Autodesk Fusion 360 part; units mm, degrees
(part 9 of 18)
  line L6113 (198.6347, -76.3898) -> (199.6463, -76.3898)
  line L6114 (199.6463, -76.3898) -> (199.6463, -77.3314)
  line L6115 (198.6347, -77.3314) -> (198.6347, -76.3898)
  line L6116 (199.6463, -77.3314) -> (198.6347, -77.3314)
  line L6117 (195.3245, -57.327) -> (196.3361, -57.327)
  line L6118 (196.3361, -58.2686) -> (195.3245, -58.2686)
  line L6119 (195.3245, -58.2686) -> (195.3245, -57.327)
  line L6120 (196.3361, -57.327) -> (196.3361, -58.2686)
  line L6121 (198.6347, -57.327) -> (199.6463, -57.327)
  line L6122 (199.6463, -58.2686) -> (198.6347, -58.2686)
  line L6123 (198.6347, -58.2686) -> (198.6347, -57.327)
  line L6124 (199.6463, -57.327) -> (199.6463, -58.2686)
  line L6125 (196.3361, -19.2142) -> (196.3361, -20.1558)
  line L6126 (195.3245, -20.1558) -> (195.3245, -19.2142)
  line L6127 (196.3361, -20.1558) -> (195.3245, -20.1558)
  line L6128 (195.3245, -19.2142) -> (196.3361, -19.2142)
  line L6129 (198.6347, -20.1558) -> (198.6347, -19.2142)
  line L6130 (199.6463, -19.2142) -> (199.6463, -20.1558)
  line L6131 (199.6463, -20.1558) -> (198.6347, -20.1558)
  line L6132 (198.6347, -19.2142) -> (199.6463, -19.2142)
  line L6133 (202.1892, -3.3092) -> (202.1892, -4.3108)
  line L6134 (201.2876, -4.3108) -> (201.2876, -3.3092)
  line L6135 (201.2876, -3.3092) -> (202.1892, -3.3092)
  line L6136 (202.1892, -4.3108) -> (201.2876, -4.3108)
  line L6137 (203.5892, -4.3108) -> (202.6876, -4.3108)
  line L6138 (202.6876, -4.3108) -> (202.6876, -3.3092)
  line L6139 (202.6876, -3.3092) -> (203.5892, -3.3092)
  line L6140 (203.5892, -3.3092) -> (203.5892, -4.3108)
  line L6141 (199.3826, -7.2318) -> (199.3826, -6.2302)
  line L6142 (200.2842, -7.2318) -> (199.3826, -7.2318)
  line L6143 (200.2842, -6.2302) -> (200.2842, -7.2318)
  line L6144 (199.3826, -6.2302) -> (200.2842, -6.2302)
  line L6145 (201.6842, -6.2302) -> (201.6842, -7.2318)
  line L6146 (201.6842, -7.2318) -> (200.7826, -7.2318)
  line L6147 (200.7826, -6.2302) -> (201.6842, -6.2302)
  line L6148 (200.7826, -7.2318) -> (200.7826, -6.2302)
  line L6149 (205.9896, -5.3268) -> (205.9896, -4.3252)
  line L6150 (206.8912, -4.3252) -> (206.8912, -5.3268)
  line L6151 (205.9896, -4.3252) -> (206.8912, -4.3252)
  line L6152 (206.8912, -5.3268) -> (205.9896, -5.3268)
  line L6153 (205.4912, -4.3252) -> (205.4912, -5.3268)
  line L6154 (204.5896, -4.3252) -> (205.4912, -4.3252)
  line L6155 (204.5896, -5.3268) -> (204.5896, -4.3252)
  line L6156 (205.4912, -5.3268) -> (204.5896, -5.3268)
  arc A664 (8.7123, -8.0011) -> (10.6139, -8.0011) centre (9.6631, -8.0011) ccw
  line L6157 (10.6139, -8.0011) -> (10.6139, -8.0011)
  arc A665 (10.6139, -8.0011) -> (8.7123, -8.0011) centre (9.6631, -8.0011) ccw
  arc A666 (8.7123, -5.4611) -> (10.6139, -5.4611) centre (9.6631, -5.4611) ccw
  arc A667 (10.6139, -5.4611) -> (8.7123, -5.4611) centre (9.6631, -5.4611) ccw
  line L6158 (10.6139, -5.4611) -> (10.6139, -5.4611)
  arc A668 (8.7123, -2.9211) -> (10.6139, -2.9211) centre (9.6631, -2.9211) ccw
  line L6159 (10.6139, -2.9211) -> (10.6139, -2.9211)
  arc A669 (10.6139, -2.9211) -> (8.7123, -2.9211) centre (9.6631, -2.9211) ccw
  arc A670 (-5.7879, -8.0011) -> (-3.8863, -8.0011) centre (-4.8371, -8.0011) ccw
  arc A671 (-3.8863, -8.0011) -> (-5.7879, -8.0011) centre (-4.8371, -8.0011) ccw
  arc A672 (-3.8863, -2.9211) -> (-5.7879, -2.9211) centre (-4.8371, -2.9211) ccw
  arc A673 (-5.7879, -2.9211) -> (-3.8863, -2.9211) centre (-4.8371, -2.9211) ccw
  line L6160 (1.3129, 1.2398) -> (3.0129, 1.2398)
  line L6161 (4.1223, -0.4205) -> (3.862, -0.8101)
  line L6162 (3.4725, 1.1484) -> (3.862, 0.8881)
  line L6163 (4.2137, 0.039) -> (4.1223, -0.4205)
  line L6164 (3.4725, -1.0704) -> (3.0129, -1.1618)
  line L6165 (0.1121, 0.039) -> (0.2035, 0.4985)
  line L6166 (0.8534, 1.1484) -> (1.3129, 1.2398)
  line L6167 (3.862, -0.8101) -> (3.4725, -1.0704)
  line L6168 (0.4638, -0.8101) -> (0.2035, -0.4205)
  line L6169 (0.4638, 0.8881) -> (0.8534, 1.1484)
  line L6170 (1.3129, -1.1618) -> (0.8534, -1.0704)
  line L6171 (0.2035, 0.4985) -> (0.4638, 0.8881)
  line L6172 (3.0129, -1.1618) -> (1.3129, -1.1618)
  line L6173 (3.0129, 1.2398) -> (3.4725, 1.1484)
  line L6174 (0.2035, -0.4205) -> (0.1121, 0.039)
  line L6175 (4.1223, 0.4985) -> (4.2137, 0.039)
  line L6176 (0.8534, -1.0704) -> (0.4638, -0.8101)
  line L6177 (3.862, 0.8881) -> (4.1223, 0.4985)
  line L6178 (3.4725, -9.8516) -> (3.862, -10.1119)
  line L6179 (1.3129, -9.7602) -> (3.0129, -9.7602)
  line L6180 (0.4638, -10.1119) -> (0.8534, -9.8516)
  line L6181 (3.0129, -12.1618) -> (1.3129, -12.1618)
  line L6182 (0.1121, -10.961) -> (0.2035, -10.5015)
  line L6183 (3.862, -10.1119) -> (4.1223, -10.5015)
  line L6184 (4.2137, -10.961) -> (4.1223, -11.4205)
  line L6185 (0.4638, -11.8101) -> (0.2035, -11.4205)
  line L6186 (4.1223, -10.5015) -> (4.2137, -10.961)
  line L6187 (3.4725, -12.0704) -> (3.0129, -12.1618)
  line L6188 (3.0129, -9.7602) -> (3.4725, -9.8516)
  line L6189 (1.3129, -12.1618) -> (0.8534, -12.0704)
  line L6190 (4.1223, -11.4205) -> (3.862, -11.8101)
  line L6191 (3.862, -11.8101) -> (3.4725, -12.0704)
  line L6192 (0.2035, -11.4205) -> (0.1121, -10.961)
  line L6193 (0.8534, -12.0704) -> (0.4638, -11.8101)
  line L6194 (0.2035, -10.5015) -> (0.4638, -10.1119)
  line L6195 (0.8534, -9.8516) -> (1.3129, -9.7602)
  line L6196 (195.6432, -3.5442) -> (195.6432, -4.0458)
  line L6197 (195.6432, -4.0458) -> (194.7416, -4.0458)
  line L6198 (194.7416, -3.5442) -> (195.6432, -3.5442)
  line L6199 (194.7416, -4.0458) -> (194.7416, -3.5442)
  line L6200 (195.6432, -4.6958) -> (194.7416, -4.6958)
  line L6201 (194.7416, -4.6958) -> (194.7416, -4.1942)
  line L6202 (194.7416, -4.1942) -> (195.6432, -4.1942)
  line L6203 (195.6432, -4.1942) -> (195.6432, -4.6958)
  line L6204 (194.7416, -5.3458) -> (194.7416, -4.8442)
  line L6205 (195.6432, -5.3458) -> (194.7416, -5.3458)
  line L6206 (194.7416, -4.8442) -> (195.6432, -4.8442)
  line L6207 (195.6432, -4.8442) -> (195.6432, -5.3458)
  line L6208 (197.0416, -4.8442) -> (197.9432, -4.8442)
  line L6209 (197.9432, -4.8442) -> (197.9432, -5.3458)
  line L6210 (197.0416, -5.3458) -> (197.0416, -4.8442)
  line L6211 (197.9432, -5.3458) -> (197.0416, -5.3458)
  line L6212 (197.9432, -4.0458) -> (197.0416, -4.0458)
  line L6213 (197.0416, -3.5442) -> (197.9432, -3.5442)
  line L6214 (197.0416, -4.0458) -> (197.0416, -3.5442)
  line L6215 (197.9432, -3.5442) -> (197.9432, -4.0458)
  arc A674 (194.7466, -61.2644) -> (196.0482, -61.2644) centre (195.3974, -61.2644) ccw
  arc A675 (196.0482, -61.2644) -> (194.7466, -61.2644) centre (195.3974, -61.2644) ccw
  arc A676 (192.5482, -63.5184) -> (191.2466, -63.5184) centre (191.8974, -63.5184) ccw
  arc A677 (191.2466, -63.5184) -> (192.5482, -63.5184) centre (191.8974, -63.5184) ccw
  arc A678 (176.9982, -80.3272) -> (175.6966, -80.3272) centre (176.3474, -80.3272) ccw
  arc A679 (175.6966, -80.3272) -> (176.9982, -80.3272) centre (176.3474, -80.3272) ccw
  arc A680 (172.1965, -82.5812) -> (173.4981, -82.5812) centre (172.8473, -82.5812) ccw
  arc A681 (173.4981, -82.5812) -> (172.1965, -82.5812) centre (172.8473, -82.5812) ccw
  arc A682 (175.6966, -61.2644) -> (176.9982, -61.2644) centre (176.3474, -61.2644) ccw
  arc A683 (176.9982, -61.2644) -> (175.6966, -61.2644) centre (176.3474, -61.2644) ccw
  arc A684 (172.1965, -63.5184) -> (173.4981, -63.5184) centre (172.8473, -63.5184) ccw
  arc A685 (173.4981, -63.5184) -> (172.1965, -63.5184) centre (172.8473, -63.5184) ccw
  arc A686 (176.9982, -42.2017) -> (175.6966, -42.2017) centre (176.3474, -42.2017) ccw
  arc A687 (175.6966, -42.2017) -> (176.9982, -42.2017) centre (176.3474, -42.2017) ccw
  arc A688 (172.1965, -44.4557) -> (173.4981, -44.4557) centre (172.8473, -44.4557) ccw
  arc A689 (173.4981, -44.4557) -> (172.1965, -44.4557) centre (172.8473, -44.4557) ccw
  arc A690 (175.6966, -23.1516) -> (176.9982, -23.1516) centre (176.3474, -23.1516) ccw
  arc A691 (176.9982, -23.1516) -> (175.6966, -23.1516) centre (176.3474, -23.1516) ccw
  arc A692 (172.1965, -25.4057) -> (173.4981, -25.4057) centre (172.8473, -25.4057) ccw
  arc A693 (173.4981, -25.4057) -> (172.1965, -25.4057) centre (172.8473, -25.4057) ccw
  arc A694 (157.9481, -80.3272) -> (156.6465, -80.3272) centre (157.2973, -80.3272) ccw
  arc A695 (156.6465, -80.3272) -> (157.9481, -80.3272) centre (157.2973, -80.3272) ccw
  arc A696 (154.4481, -82.5812) -> (153.1465, -82.5812) centre (153.7973, -82.5812) ccw
  arc A697 (153.1465, -82.5812) -> (154.4481, -82.5812) centre (153.7973, -82.5812) ccw
  arc A698 (157.9481, -42.2017) -> (156.6465, -42.2017) centre (157.2973, -42.2017) ccw
  arc A699 (156.6465, -42.2017) -> (157.9481, -42.2017) centre (157.2973, -42.2017) ccw
  arc A700 (153.1465, -44.4557) -> (154.4481, -44.4557) centre (153.7973, -44.4557) ccw
  arc A701 (154.4481, -44.4557) -> (153.1465, -44.4557) centre (153.7973, -44.4557) ccw
  arc A702 (157.9481, -61.2644) -> (156.6465, -61.2644) centre (157.2973, -61.2644) ccw
  arc A703 (156.6465, -61.2644) -> (157.9481, -61.2644) centre (157.2973, -61.2644) ccw
  arc A704 (153.1465, -63.5184) -> (154.4481, -63.5184) centre (153.7973, -63.5184) ccw
  arc A705 (154.4481, -63.5184) -> (153.1465, -63.5184) centre (153.7973, -63.5184) ccw
  arc A706 (156.6465, -23.1516) -> (157.9481, -23.1516) centre (157.2973, -23.1516) ccw
  arc A707 (157.9481, -23.1516) -> (156.6465, -23.1516) centre (157.2973, -23.1516) ccw
  arc A708 (154.4481, -25.4057) -> (153.1465, -25.4057) centre (153.7973, -25.4057) ccw
  arc A709 (153.1465, -25.4057) -> (154.4481, -25.4057) centre (153.7973, -25.4057) ccw
  arc A710 (137.5965, -61.2644) -> (138.8981, -61.2644) centre (138.2473, -61.2644) ccw
  arc A711 (138.8981, -61.2644) -> (137.5965, -61.2644) centre (138.2473, -61.2644) ccw
  arc A712 (135.3981, -63.5184) -> (134.0965, -63.5184) centre (134.7473, -63.5184) ccw
  arc A713 (134.0965, -63.5184) -> (135.3981, -63.5184) centre (134.7473, -63.5184) ccw
  arc A714 (137.5965, -42.2017) -> (138.8981, -42.2017) centre (138.2473, -42.2017) ccw
  arc A715 (138.8981, -42.2017) -> (137.5965, -42.2017) centre (138.2473, -42.2017) ccw
  arc A716 (134.0965, -44.4557) -> (135.3981, -44.4557) centre (134.7473, -44.4557) ccw
  arc A717 (135.3981, -44.4557) -> (134.0965, -44.4557) centre (134.7473, -44.4557) ccw
  arc A718 (138.8981, -23.1516) -> (137.5965, -23.1516) centre (138.2473, -23.1516) ccw
  arc A719 (137.5965, -23.1516) -> (138.8981, -23.1516) centre (138.2473, -23.1516) ccw
  arc A720 (134.0965, -25.4057) -> (135.3981, -25.4057) centre (134.7473, -25.4057) ccw
  arc A721 (135.3981, -25.4057) -> (134.0965, -25.4057) centre (134.7473, -25.4057) ccw
  arc A722 (137.5965, -80.3272) -> (138.8981, -80.3272) centre (138.2473, -80.3272) ccw
  arc A723 (138.8981, -80.3272) -> (137.5965, -80.3272) centre (138.2473, -80.3272) ccw
  arc A724 (135.3981, -82.5812) -> (134.0965, -82.5812) centre (134.7473, -82.5812) ccw
  arc A725 (134.0965, -82.5812) -> (135.3981, -82.5812) centre (134.7473, -82.5812) ccw
  arc A726 (119.848, -80.3272) -> (118.5464, -80.3272) centre (119.1972, -80.3272) ccw
  arc A727 (118.5464, -80.3272) -> (119.848, -80.3272) centre (119.1972, -80.3272) ccw
  arc A728 (115.0464, -82.5812) -> (116.348, -82.5812) centre (115.6972, -82.5812) ccw
  arc A729 (116.348, -82.5812) -> (115.0464, -82.5812) centre (115.6972, -82.5812) ccw
  arc A730 (118.5464, -61.2644) -> (119.848, -61.2644) centre (119.1972, -61.2644) ccw
  arc A731 (119.848, -61.2644) -> (118.5464, -61.2644) centre (119.1972, -61.2644) ccw
  arc A732 (115.0464, -63.5184) -> (116.348, -63.5184) centre (115.6972, -63.5184) ccw
  arc A733 (116.348, -63.5184) -> (115.0464, -63.5184) centre (115.6972, -63.5184) ccw
  arc A734 (118.5464, -23.1516) -> (119.848, -23.1516) centre (119.1972, -23.1516) ccw
  arc A735 (119.848, -23.1516) -> (118.5464, -23.1516) centre (119.1972, -23.1516) ccw
  arc A736 (115.0464, -25.4057) -> (116.348, -25.4057) centre (115.6972, -25.4057) ccw
  arc A737 (116.348, -25.4057) -> (115.0464, -25.4057) centre (115.6972, -25.4057) ccw
  arc A738 (119.848, -42.2017) -> (118.5464, -42.2017) centre (119.1972, -42.2017) ccw
  arc A739 (118.5464, -42.2017) -> (119.848, -42.2017) centre (119.1972, -42.2017) ccw
  arc A740 (116.348, -44.4557) -> (115.0464, -44.4557) centre (115.6972, -44.4557) ccw
  arc A741 (115.0464, -44.4557) -> (116.348, -44.4557) centre (115.6972, -44.4557) ccw
  arc A742 (100.798, -23.1516) -> (99.4964, -23.1516) centre (100.1472, -23.1516) ccw
  arc A743 (99.4964, -23.1516) -> (100.798, -23.1516) centre (100.1472, -23.1516) ccw
  arc A744 (95.9964, -25.4057) -> (97.298, -25.4057) centre (96.6472, -25.4057) ccw
  arc A745 (97.298, -25.4057) -> (95.9964, -25.4057) centre (96.6472, -25.4057) ccw
  arc A746 (100.798, -42.2017) -> (99.4964, -42.2017) centre (100.1472, -42.2017) ccw
  arc A747 (99.4964, -42.2017) -> (100.798, -42.2017) centre (100.1472, -42.2017) ccw
  arc A748 (97.298, -44.4557) -> (95.9964, -44.4557) centre (96.6472, -44.4557) ccw
  arc A749 (95.9964, -44.4557) -> (97.298, -44.4557) centre (96.6472, -44.4557) ccw
  arc A750 (100.798, -80.3272) -> (99.4964, -80.3272) centre (100.1472, -80.3272) ccw
  arc A751 (99.4964, -80.3272) -> (100.798, -80.3272) centre (100.1472, -80.3272) ccw
  arc A752 (95.9964, -82.5812) -> (97.298, -82.5812) centre (96.6472, -82.5812) ccw
  arc A753 (97.298, -82.5812) -> (95.9964, -82.5812) centre (96.6472, -82.5812) ccw
  arc A754 (100.798, -61.2644) -> (99.4964, -61.2644) centre (100.1472, -61.2644) ccw
  arc A755 (99.4964, -61.2644) -> (100.798, -61.2644) centre (100.1472, -61.2644) ccw
  arc A756 (97.298, -63.5184) -> (95.9964, -63.5184) centre (96.6472, -63.5184) ccw
  arc A757 (95.9964, -63.5184) -> (97.298, -63.5184) centre (96.6472, -63.5184) ccw
  arc A758 (194.7466, -80.3272) -> (196.0482, -80.3272) centre (195.3974, -80.3272) ccw
  arc A759 (196.0482, -80.3272) -> (194.7466, -80.3272) centre (195.3974, -80.3272) ccw
  arc A760 (192.5482, -82.5812) -> (191.2466, -82.5812) centre (191.8974, -82.5812) ccw
  arc A761 (191.2466, -82.5812) -> (192.5482, -82.5812) centre (191.8974, -82.5812) ccw
  arc A762 (194.7466, -23.1516) -> (196.0482, -23.1516) centre (195.3974, -23.1516) ccw
  arc A763 (196.0482, -23.1516) -> (194.7466, -23.1516) centre (195.3974, -23.1516) ccw
  arc A764 (191.2466, -25.4057) -> (192.5482, -25.4057) centre (191.8974, -25.4057) ccw
  arc A765 (192.5482, -25.4057) -> (191.2466, -25.4057) centre (191.8974, -25.4057) ccw
  arc A766 (80.4464, -80.3272) -> (81.748, -80.3272) centre (81.0972, -80.3272) ccw
  arc A767 (81.748, -80.3272) -> (80.4464, -80.3272) centre (81.0972, -80.3272) ccw
  arc A768 (76.9464, -82.5812) -> (78.248, -82.5812) centre (77.5972, -82.5812) ccw
  arc A769 (78.248, -82.5812) -> (76.9464, -82.5812) centre (77.5972, -82.5812) ccw
  arc A770 (80.4464, -42.2017) -> (81.748, -42.2017) centre (81.0972, -42.2017) ccw
  arc A771 (81.748, -42.2017) -> (80.4464, -42.2017) centre (81.0972, -42.2017) ccw
  arc A772 (78.248, -44.4557) -> (76.9464, -44.4557) centre (77.5972, -44.4557) ccw
  arc A773 (76.9464, -44.4557) -> (78.248, -44.4557) centre (77.5972, -44.4557) ccw
  arc A774 (80.4464, -23.1516) -> (81.748, -23.1516) centre (81.0972, -23.1516) ccw
  arc A775 (81.748, -23.1516) -> (80.4464, -23.1516) centre (81.0972, -23.1516) ccw
  arc A776 (78.248, -25.4057) -> (76.9464, -25.4057) centre (77.5972, -25.4057) ccw
  arc A777 (76.9464, -25.4057) -> (78.248, -25.4057) centre (77.5972, -25.4057) ccw
  arc A778 (80.4464, -61.2644) -> (81.748, -61.2644) centre (81.0972, -61.2644) ccw
  arc A779 (81.748, -61.2644) -> (80.4464, -61.2644) centre (81.0972, -61.2644) ccw
  arc A780 (78.248, -63.5184) -> (76.9464, -63.5184) centre (77.5972, -63.5184) ccw
  arc A781 (76.9464, -63.5184) -> (78.248, -63.5184) centre (77.5972, -63.5184) ccw
  arc A782 (61.3963, -80.3272) -> (62.6979, -80.3272) centre (62.0471, -80.3272) ccw
  arc A783 (62.6979, -80.3272) -> (61.3963, -80.3272) centre (62.0471, -80.3272) ccw
  arc A784 (59.1979, -82.5812) -> (57.8963, -82.5812) centre (58.5471, -82.5812) ccw
  arc A785 (57.8963, -82.5812) -> (59.1979, -82.5812) centre (58.5471, -82.5812) ccw
  arc A786 (61.3963, -61.2644) -> (62.6979, -61.2644) centre (62.0471, -61.2644) ccw
  arc A787 (62.6979, -61.2644) -> (61.3963, -61.2644) centre (62.0471, -61.2644) ccw
  arc A788 (57.8963, -63.5184) -> (59.1979, -63.5184) centre (58.5471, -63.5184) ccw
  arc A789 (59.1979, -63.5184) -> (57.8963, -63.5184) centre (58.5471, -63.5184) ccw
  arc A790 (62.6979, -42.2017) -> (61.3963, -42.2017) centre (62.0471, -42.2017) ccw
  arc A791 (61.3963, -42.2017) -> (62.6979, -42.2017) centre (62.0471, -42.2017) ccw
  arc A792 (59.1979, -44.4557) -> (57.8963, -44.4557) centre (58.5471, -44.4557) ccw
  arc A793 (57.8963, -44.4557) -> (59.1979, -44.4557) centre (58.5471, -44.4557) ccw
  arc A794 (43.6479, -61.2644) -> (42.3463, -61.2644) centre (42.9971, -61.2644) ccw
  arc A795 (42.3463, -61.2644) -> (43.6479, -61.2644) centre (42.9971, -61.2644) ccw
  arc A796 (38.8463, -63.5184) -> (40.1479, -63.5184) centre (39.4971, -63.5184) ccw
  arc A797 (40.1479, -63.5184) -> (38.8463, -63.5184) centre (39.4971, -63.5184) ccw
  arc A798 (43.6479, -80.3272) -> (42.3463, -80.3272) centre (42.9971, -80.3272) ccw
  arc A799 (42.3463, -80.3272) -> (43.6479, -80.3272) centre (42.9971, -80.3272) ccw
  arc A800 (40.1479, -82.5812) -> (38.8463, -82.5812) centre (39.4971, -82.5812) ccw
  arc A801 (38.8463, -82.5812) -> (40.1479, -82.5812) centre (39.4971, -82.5812) ccw
  arc A802 (24.5978, -80.3272) -> (23.2962, -80.3272) centre (23.947, -80.3272) ccw
  arc A803 (23.2962, -80.3272) -> (24.5978, -80.3272) centre (23.947, -80.3272) ccw
  arc A804 (19.7962, -82.5812) -> (21.0978, -82.5812) centre (20.447, -82.5812) ccw
  arc A805 (21.0978, -82.5812) -> (19.7962, -82.5812) centre (20.447, -82.5812) ccw
  arc A806 (5.5478, -80.3272) -> (4.2462, -80.3272) centre (4.897, -80.3272) ccw
  arc A807 (4.2462, -80.3272) -> (5.5478, -80.3272) centre (4.897, -80.3272) ccw
  arc A808 (2.0478, -82.5812) -> (0.7462, -82.5812) centre (1.397, -82.5812) ccw
  arc A809 (0.7462, -82.5812) -> (2.0478, -82.5812) centre (1.397, -82.5812) ccw
  arc A810 (61.3963, -23.1516) -> (62.6979, -23.1516) centre (62.0471, -23.1516) ccw
  arc A811 (62.6979, -23.1516) -> (61.3963, -23.1516) centre (62.0471, -23.1516) ccw
  arc A812 (59.1979, -25.4057) -> (57.8963, -25.4057) centre (58.5471, -25.4057) ccw
  arc A813 (57.8963, -25.4057) -> (59.1979, -25.4057) centre (58.5471, -25.4057) ccw
  arc A814 (43.6479, -42.2017) -> (42.3463, -42.2017) centre (42.9971, -42.2017) ccw
  arc A815 (42.3463, -42.2017) -> (43.6479, -42.2017) centre (42.9971, -42.2017) ccw
  arc A816 (40.1479, -44.4557) -> (38.8463, -44.4557) centre (39.4971, -44.4557) ccw
  arc A817 (38.8463, -44.4557) -> (40.1479, -44.4557) centre (39.4971, -44.4557) ccw
  arc A818 (43.6479, -23.1516) -> (42.3463, -23.1516) centre (42.9971, -23.1516) ccw
  arc A819 (42.3463, -23.1516) -> (43.6479, -23.1516) centre (42.9971, -23.1516) ccw
  arc A820 (40.1479, -25.4057) -> (38.8463, -25.4057) centre (39.4971, -25.4057) ccw
  arc A821 (38.8463, -25.4057) -> (40.1479, -25.4057) centre (39.4971, -25.4057) ccw
  arc A822 (23.2962, -23.1516) -> (24.5978, -23.1516) centre (23.947, -23.1516) ccw
  arc A823 (24.5978, -23.1516) -> (23.2962, -23.1516) centre (23.947, -23.1516) ccw
  arc A824 (19.7962, -25.4057) -> (21.0978, -25.4057) centre (20.447, -25.4057) ccw
  arc A825 (21.0978, -25.4057) -> (19.7962, -25.4057) centre (20.447, -25.4057) ccw
  arc A826 (24.5978, -61.2644) -> (23.2962, -61.2644) centre (23.947, -61.2644) ccw
  arc A827 (23.2962, -61.2644) -> (24.5978, -61.2644) centre (23.947, -61.2644) ccw
  arc A828 (21.0978, -63.5184) -> (19.7962, -63.5184) centre (20.447, -63.5184) ccw
  arc A829 (19.7962, -63.5184) -> (21.0978, -63.5184) centre (20.447, -63.5184) ccw
  arc A830 (24.5978, -42.2017) -> (23.2962, -42.2017) centre (23.947, -42.2017) ccw
  arc A831 (23.2962, -42.2017) -> (24.5978, -42.2017) centre (23.947, -42.2017) ccw
  arc A832 (21.0978, -44.4557) -> (19.7962, -44.4557) centre (20.447, -44.4557) ccw
  arc A833 (19.7962, -44.4557) -> (21.0978, -44.4557) centre (20.447, -44.4557) ccw
  arc A834 (5.5478, -23.1516) -> (4.2462, -23.1516) centre (4.897, -23.1516) ccw
  arc A835 (4.2462, -23.1516) -> (5.5478, -23.1516) centre (4.897, -23.1516) ccw
  arc A836 (0.7462, -25.4057) -> (2.0478, -25.4057) centre (1.397, -25.4057) ccw
  arc A837 (2.0478, -25.4057) -> (0.7462, -25.4057) centre (1.397, -25.4057) ccw
  arc A838 (5.5478, -42.2017) -> (4.2462, -42.2017) centre (4.897, -42.2017) ccw
  arc A839 (4.2462, -42.2017) -> (5.5478, -42.2017) centre (4.897, -42.2017) ccw
  arc A840 (2.0478, -44.4557) -> (0.7462, -44.4557) centre (1.397, -44.4557) ccw
  arc A841 (0.7462, -44.4557) -> (2.0478, -44.4557) centre (1.397, -44.4557) ccw
  arc A842 (4.2462, -61.2644) -> (5.5478, -61.2644) centre (4.897, -61.2644) ccw
  arc A843 (5.5478, -61.2644) -> (4.2462, -61.2644) centre (4.897, -61.2644) ccw
  arc A844 (2.0478, -63.5184) -> (0.7462, -63.5184) centre (1.397, -63.5184) ccw
  arc A845 (0.7462, -63.5184) -> (2.0478, -63.5184) centre (1.397, -63.5184) ccw
  arc A846 (213.7966, -61.2644) -> (215.0982, -61.2644) centre (214.4474, -61.2644) ccw
  arc A847 (215.0982, -61.2644) -> (213.7966, -61.2644) centre (214.4474, -61.2644) ccw
  arc A848 (211.5982, -63.5184) -> (210.2966, -63.5184) centre (210.9474, -63.5184) ccw
  arc A849 (210.2966, -63.5184) -> (211.5982, -63.5184) centre (210.9474, -63.5184) ccw
  arc A850 (215.0982, -42.2017) -> (213.7966, -42.2017) centre (214.4474, -42.2017) ccw
  arc A851 (213.7966, -42.2017) -> (215.0982, -42.2017) centre (214.4474, -42.2017) ccw
  arc A852 (210.2966, -44.4557) -> (211.5982, -44.4557) centre (210.9474, -44.4557) ccw
  arc A853 (211.5982, -44.4557) -> (210.2966, -44.4557) centre (210.9474, -44.4557) ccw
  arc A854 (215.0982, -23.1516) -> (213.7966, -23.1516) centre (214.4474, -23.1516) ccw
  arc A855 (213.7966, -23.1516) -> (215.0982, -23.1516) centre (214.4474, -23.1516) ccw
  arc A856 (211.5982, -25.4057) -> (210.2966, -25.4057) centre (210.9474, -25.4057) ccw
  arc A857 (210.2966, -25.4057) -> (211.5982, -25.4057) centre (210.9474, -25.4057) ccw
  arc A858 (215.0982, -80.3272) -> (213.7966, -80.3272) centre (214.4474, -80.3272) ccw
  arc A859 (213.7966, -80.3272) -> (215.0982, -80.3272) centre (214.4474, -80.3272) ccw
  arc A860 (211.5982, -82.5812) -> (210.2966, -82.5812) centre (210.9474, -82.5812) ccw
  arc A861 (210.2966, -82.5812) -> (211.5982, -82.5812) centre (210.9474, -82.5812) ccw
  arc A862 (194.7466, -42.2017) -> (196.0482, -42.2017) centre (195.3974, -42.2017) ccw
  arc A863 (196.0482, -42.2017) -> (194.7466, -42.2017) centre (195.3974, -42.2017) ccw
  arc A864 (191.2466, -44.4557) -> (192.5482, -44.4557) centre (191.8974, -44.4557) ccw
  arc A865 (192.5482, -44.4557) -> (191.2466, -44.4557) centre (191.8974, -44.4557) ccw
  arc A866 (176.9732, -4.318) -> (175.0716, -4.318) centre (176.0224, -4.318) ccw
  arc A867 (175.0716, -4.318) -> (176.9732, -4.318) centre (176.0224, -4.318) ccw
  line L6216 (172.5315, -5.2688) -> (172.5315, -3.3672)
  line L6217 (172.5315, -3.3672) -> (174.4331, -3.3672)
  line L6218 (174.4331, -5.2688) -> (172.5315, -5.2688)
  line L6219 (174.4331, -3.3672) -> (174.4331, -5.2688)
  line L6220 (200.2654, -1.455) -> (199.4654, -1.455)
  line L6221 (200.3154, -2.305) -> (200.3154, -2.077)
  line L6222 (199.4654, -1.455) -> (199.4154, -1.505)
  line L6223 (199.4654, -2.355) -> (200.2654, -2.355)
  line L6224 (199.9454, -2.077) -> (199.9454, -1.747)
  line L6225 (199.4154, -1.505) -> (199.4154, -2.305)
  line L6226 (200.3154, -1.747) -> (200.3154, -1.505)
  line L6227 (199.4154, -2.305) -> (199.4654, -2.355)
  line L6228 (199.9454, -1.747) -> (200.3154, -1.747)
  line L6229 (200.3154, -2.077) -> (199.9454, -2.077)
  line L6230 (200.2654, -2.355) -> (200.3154, -2.305)
  line L6231 (200.3154, -1.505) -> (200.2654, -1.455)
  line L6232 (201.0554, -2.355) -> (201.8554, -2.355)
  line L6233 (201.3754, -1.733) -> (201.3754, -2.063)
  line L6234 (201.8554, -2.355) -> (201.9054, -2.305)
  line L6235 (201.0054, -2.063) -> (201.0054, -2.305)
  line L6236 (201.0554, -1.455) -> (201.0054, -1.505)
  line L6237 (201.3754, -2.063) -> (201.0054, -2.063)
  line L6238 (201.0054, -1.505) -> (201.0054, -1.733)
  line L6239 (201.9054, -1.505) -> (201.8554, -1.455)
  line L6240 (201.0054, -2.305) -> (201.0554, -2.355)
  line L6241 (201.9054, -2.305) -> (201.9054, -1.505)
  line L6242 (201.0054, -1.733) -> (201.3754, -1.733)
  line L6243 (201.8554, -1.455) -> (201.0554, -1.455)
  line L6244 (208.3746, -5.023) -> (208.3746, -5.688)
  line L6245 (208.5746, -5.688) -> (208.5746, -5.023)
  line L6246 (208.3746, -5.688) -> (208.5746, -5.688)
  line L6247 (208.5746, -5.023) -> (208.3746, -5.023)
  line L6248 (211.3744, -5.688) -> (211.3744, -5.023)
  line L6249 (211.1744, -5.688) -> (211.3744, -5.688)
  line L6250 (211.1744, -5.023) -> (211.1744, -5.688)
  line L6251 (211.3744, -5.023) -> (211.1744, -5.023)
  line L6252 (210.7744, -5.023) -> (210.7744, -5.688)
  line L6253 (210.9744, -5.688) -> (210.9744, -5.023)
  line L6254 (210.7744, -5.688) -> (210.9744, -5.688)
  line L6255 (210.9744, -5.023) -> (210.7744, -5.023)
  line L6256 (213.5745, -5.688) -> (213.7745, -5.688)
  line L6257 (213.7745, -5.688) -> (213.7745, -5.023)
  line L6258 (213.5745, -5.023) -> (213.5745, -5.688)
  line L6259 (213.7745, -5.023) -> (213.5745, -5.023)
  line L6260 (208.9744, -5.688) -> (208.9744, -5.023)
  line L6261 (208.7744, -5.688) -> (208.9744, -5.688)
  line L6262 (208.9744, -5.023) -> (208.7744, -5.023)
  line L6263 (208.7744, -5.023) -> (208.7744, -5.688)
  line L6264 (211.7745, -5.023) -> (211.5745, -5.023)
  line L6265 (211.7745, -5.688) -> (211.7745, -5.023)
  line L6266 (211.5745, -5.688) -> (211.7745, -5.688)
  line L6267 (211.5745, -5.023) -> (211.5745, -5.688)
  line L6268 (209.1744, -5.688) -> (209.3744, -5.688)
  line L6269 (209.3744, -5.023) -> (209.1744, -5.023)
  line L6270 (209.3744, -5.688) -> (209.3744, -5.023)
  line L6271 (209.1744, -5.023) -> (209.1744, -5.688)
  line L6272 (211.9745, -5.688) -> (212.1745, -5.688)
  line L6273 (211.9745, -5.023) -> (211.9745, -5.688)
  line L6274 (212.1745, -5.688) -> (212.1745, -5.023)
  line L6275 (212.1745, -5.023) -> (211.9745, -5.023)
  line L6276 (209.5745, -5.023) -> (209.5745, -5.688)
  line L6277 (209.7745, -5.023) -> (209.5745, -5.023)
  line L6278 (209.5745, -5.688) -> (209.7745, -5.688)
  line L6279 (209.7745, -5.688) -> (209.7745, -5.023)
  line L6280 (212.5746, -5.688) -> (212.5746, -5.023)
  line L6281 (212.3746, -5.688) -> (212.5746, -5.688)
  line L6282 (212.3746, -5.023) -> (212.3746, -5.688)
  line L6283 (212.5746, -5.023) -> (212.3746, -5.023)
  line L6284 (210.5746, -5.023) -> (210.3746, -5.023)
  line L6285 (210.3746, -5.688) -> (210.5746, -5.688)
  line L6286 (210.3746, -5.023) -> (210.3746, -5.688)
  line L6287 (210.5746, -5.688) -> (210.5746, -5.023)
  line L6288 (213.1744, -5.688) -> (213.3744, -5.688)
  line L6289 (213.3744, -5.023) -> (213.1744, -5.023)
  line L6290 (213.1744, -5.023) -> (213.1744, -5.688)
  line L6291 (213.3744, -5.688) -> (213.3744, -5.023)
  line L6292 (210.1745, -5.688) -> (210.1745, -5.023)
  line L6293 (210.1745, -5.023) -> (209.9745, -5.023)
  line L6294 (209.9745, -5.023) -> (209.9745, -5.688)
  line L6295 (209.9745, -5.688) -> (210.1745, -5.688)
  line L6296 (212.7744, -5.023) -> (212.7744, -5.688)
  line L6297 (212.9744, -5.688) -> (212.9744, -5.023)
  line L6298 (212.9744, -5.023) -> (212.7744, -5.023)
  line L6299 (212.7744, -5.688) -> (212.9744, -5.688)
  line L6300 (207.3344, -6.0629) -> (207.3344, -6.2629)
  line L6301 (207.9994, -6.0629) -> (207.3344, -6.0629)
  line L6302 (207.3344, -6.2629) -> (207.9994, -6.2629)
  line L6303 (207.9994, -6.2629) -> (207.9994, -6.0629)
  line L6304 (214.1495, -6.0629) -> (214.1495, -6.2629)
  line L6305 (214.8145, -6.2629) -> (214.8145, -6.0629)
  line L6306 (214.8145, -6.0629) -> (214.1495, -6.0629)
  line L6307 (214.1495, -6.2629) -> (214.8145, -6.2629)
  line L6308 (207.3344, -6.663) -> (207.9994, -6.663)
  line L6309 (207.3344, -6.463) -> (207.3344, -6.663)
  line L6310 (207.9994, -6.463) -> (207.3344, -6.463)
  line L6311 (207.9994, -6.663) -> (207.9994, -6.463)
  line L6312 (214.1495, -6.663) -> (214.8145, -6.663)
  line L6313 (214.8145, -6.463) -> (214.1495, -6.463)
  line L6314 (214.8145, -6.663) -> (214.8145, -6.463)
  line L6315 (214.1495, -6.463) -> (214.1495, -6.663)
  line L6316 (207.3344, -6.863) -> (207.3344, -7.063)
  line L6317 (207.9994, -6.863) -> (207.3344, -6.863)
  line L6318 (207.9994, -7.063) -> (207.9994, -6.863)
  line L6319 (207.3344, -7.063) -> (207.9994, -7.063)
  line L6320 (214.8145, -6.863) -> (214.1495, -6.863)
  line L6321 (214.1495, -6.863) -> (214.1495, -7.063)
  line L6322 (214.1495, -7.063) -> (214.8145, -7.063)
  line L6323 (214.8145, -7.063) -> (214.8145, -6.863)
  line L6324 (214.8145, -7.4628) -> (214.8145, -7.2628)
  line L6325 (214.1495, -7.2628) -> (214.1495, -7.4628)
  line L6326 (214.8145, -7.2628) -> (214.1495, -7.2628)
  line L6327 (214.1495, -7.4628) -> (214.8145, -7.4628)
  line L6328 (207.9994, -7.2628) -> (207.3344, -7.2628)
  line L6329 (207.3344, -7.2628) -> (207.3344, -7.4628)
  line L6330 (207.3344, -7.4628) -> (207.9994, -7.4628)
  line L6331 (207.9994, -7.4628) -> (207.9994, -7.2628)
  line L6332 (207.9994, -7.6629) -> (207.3344, -7.6629)
  line L6333 (207.3344, -7.6629) -> (207.3344, -7.8629)
  line L6334 (207.3344, -7.8629) -> (207.9994, -7.8629)
  line L6335 (207.9994, -7.8629) -> (207.9994, -7.6629)
  line L6336 (214.1495, -7.8629) -> (214.8145, -7.8629)
  line L6337 (214.8145, -7.8629) -> (214.8145, -7.6629)
  line L6338 (214.8145, -7.6629) -> (214.1495, -7.6629)
  line L6339 (214.1495, -7.6629) -> (214.1495, -7.8629)
  line L6340 (207.9994, -8.0629) -> (207.3344, -8.0629)
  line L6341 (207.3344, -8.2629) -> (207.9994, -8.2629)
  line L6342 (207.9994, -8.2629) -> (207.9994, -8.0629)
  line L6343 (207.3344, -8.0629) -> (207.3344, -8.2629)
  line L6344 (214.1495, -8.2629) -> (214.8145, -8.2629)
  line L6345 (214.8145, -8.2629) -> (214.8145, -8.0629)
  line L6346 (214.8145, -8.0629) -> (214.1495, -8.0629)
  line L6347 (214.1495, -8.0629) -> (214.1495, -8.2629)
  line L6348 (207.9994, -8.463) -> (207.3344, -8.463)
  line L6349 (207.3344, -8.463) -> (207.3344, -8.663)
  line L6350 (207.3344, -8.663) -> (207.9994, -8.663)
  line L6351 (207.9994, -8.663) -> (207.9994, -8.463)
  line L6352 (214.1495, -8.663) -> (214.8145, -8.663)
  line L6353 (214.8145, -8.663) -> (214.8145, -8.463)
  line L6354 (214.8145, -8.463) -> (214.1495, -8.463)
  line L6355 (214.1495, -8.463) -> (214.1495, -8.663)
  line L6356 (207.3344, -9.063) -> (207.9994, -9.063)
  line L6357 (207.9994, -8.863) -> (207.3344, -8.863)
  line L6358 (207.9994, -9.063) -> (207.9994, -8.863)
  line L6359 (207.3344, -8.863) -> (207.3344, -9.063)
  line L6360 (214.8145, -9.063) -> (214.8145, -8.863)
  line L6361 (214.8145, -8.863) -> (214.1495, -8.863)
  line L6362 (214.1495, -8.863) -> (214.1495, -9.063)
  line L6363 (214.1495, -9.063) -> (214.8145, -9.063)
  line L6364 (207.9994, -9.4628) -> (207.9994, -9.2628)
  line L6365 (207.9994, -9.2628) -> (207.3344, -9.2628)
  line L6366 (207.3344, -9.2628) -> (207.3344, -9.4628)
  line L6367 (207.3344, -9.4628) -> (207.9994, -9.4628)
  line L6368 (214.1495, -9.4628) -> (214.8145, -9.4628)
  line L6369 (214.1495, -9.2628) -> (214.1495, -9.4628)
  line L6370 (214.8145, -9.4628) -> (214.8145, -9.2628)
  line L6371 (214.8145, -9.2628) -> (214.1495, -9.2628)
  line L6372 (207.3344, -9.6629) -> (207.3344, -9.8629)
  line L6373 (207.9994, -9.8629) -> (207.9994, -9.6629)
  line L6374 (207.3344, -9.8629) -> (207.9994, -9.8629)
  line L6375 (207.9994, -9.6629) -> (207.3344, -9.6629)
  line L6376 (214.1495, -9.6629) -> (214.1495, -9.8629)
  line L6377 (214.8145, -9.6629) -> (214.1495, -9.6629)
  line L6378 (214.8145, -9.8629) -> (214.8145, -9.6629)
  line L6379 (214.1495, -9.8629) -> (214.8145, -9.8629)
  line L6380 (214.8145, -10.2629) -> (214.8145, -10.0629)
  line L6381 (214.8145, -10.0629) -> (214.1495, -10.0629)
  line L6382 (214.1495, -10.0629) -> (214.1495, -10.2629)
  line L6383 (214.1495, -10.2629) -> (214.8145, -10.2629)
  line L6384 (207.9994, -10.0629) -> (207.3344, -10.0629)
  line L6385 (207.9994, -10.2629) -> (207.9994, -10.0629)
  line L6386 (207.3344, -10.0629) -> (207.3344, -10.2629)
  line L6387 (207.3344, -10.2629) -> (207.9994, -10.2629)
  line L6388 (207.9994, -10.663) -> (207.9994, -10.463)
  line L6389 (207.3344, -10.463) -> (207.3344, -10.663)
  line L6390 (207.3344, -10.663) -> (207.9994, -10.663)
  line L6391 (207.9994, -10.463) -> (207.3344, -10.463)
  line L6392 (214.8145, -10.463) -> (214.1495, -10.463)
  line L6393 (214.1495, -10.463) -> (214.1495, -10.663)
  line L6394 (214.8145, -10.663) -> (214.8145, -10.463)
  line L6395 (214.1495, -10.663) -> (214.8145, -10.663)
  line L6396 (207.3344, -11.063) -> (207.9994, -11.063)
  line L6397 (207.3344, -10.863) -> (207.3344, -11.063)
  line L6398 (207.9994, -10.863) -> (207.3344, -10.863)
  line L6399 (207.9994, -11.063) -> (207.9994, -10.863)
  line L6400 (214.8145, -11.063) -> (214.8145, -10.863)
  line L6401 (214.8145, -10.863) -> (214.1495, -10.863)
  line L6402 (214.1495, -10.863) -> (214.1495, -11.063)
  line L6403 (214.1495, -11.063) -> (214.8145, -11.063)
  line L6404 (207.3344, -11.4628) -> (207.9994, -11.4628)
  line L6405 (207.9994, -11.4628) -> (207.9994, -11.2628)
  line L6406 (207.9994, -11.2628) -> (207.3344, -11.2628)
  line L6407 (207.3344, -11.2628) -> (207.3344, -11.4628)
  line L6408 (214.8145, -11.2628) -> (214.1495, -11.2628)
  line L6409 (214.1495, -11.4628) -> (214.8145, -11.4628)
  line L6410 (214.8145, -11.4628) -> (214.8145, -11.2628)
  line L6411 (214.1495, -11.2628) -> (214.1495, -11.4628)
  line L6412 (213.7745, -12.5031) -> (213.7745, -11.8381)
  line L6413 (213.7745, -11.8381) -> (213.5745, -11.8381)
  line L6414 (213.5745, -12.5031) -> (213.7745, -12.5031)
  line L6415 (213.5745, -11.8381) -> (213.5745, -12.5031)
  line L6416 (210.7744, -12.5031) -> (210.9744, -12.5031)
  line L6417 (210.9744, -12.5031) -> (210.9744, -11.8381)
  line L6418 (210.9744, -11.8381) -> (210.7744, -11.8381)
  line L6419 (210.7744, -11.8381) -> (210.7744, -12.5031)
  line L6420 (211.3744, -12.5031) -> (211.3744, -11.8381)
  line L6421 (211.1744, -11.8381) -> (211.1744, -12.5031)
  line L6422 (211.1744, -12.5031) -> (211.3744, -12.5031)
  line L6423 (211.3744, -11.8381) -> (211.1744, -11.8381)
  line L6424 (208.3746, -11.8381) -> (208.3746, -12.5031)
  line L6425 (208.5746, -12.5031) -> (208.5746, -11.8381)
  line L6426 (208.5746, -11.8381) -> (208.3746, -11.8381)
  line L6427 (208.3746, -12.5031) -> (208.5746, -12.5031)
  line L6428 (213.3744, -12.5031) -> (213.3744, -11.8381)
  line L6429 (213.1744, -11.8381) -> (213.1744, -12.5031)
  line L6430 (213.1744, -12.5031) -> (213.3744, -12.5031)
  line L6431 (213.3744, -11.8381) -> (213.1744, -11.8381)
  line L6432 (210.3746, -11.8381) -> (210.3746, -12.5031)
  line L6433 (210.3746, -12.5031) -> (210.5746, -12.5031)
  line L6434 (210.5746, -11.8381) -> (210.3746, -11.8381)
  line L6435 (210.5746, -12.5031) -> (210.5746, -11.8381)
  line L6436 (212.7744, -12.5031) -> (212.9744, -12.5031)
  line L6437 (212.7744, -11.8381) -> (212.7744, -12.5031)
  line L6438 (212.9744, -11.8381) -> (212.7744, -11.8381)
  line L6439 (212.9744, -12.5031) -> (212.9744, -11.8381)
  line L6440 (210.1745, -12.5031) -> (210.1745, -11.8381)
  line L6441 (209.9745, -11.8381) -> (209.9745, -12.5031)
  line L6442 (210.1745, -11.8381) -> (209.9745, -11.8381)
  line L6443 (209.9745, -12.5031) -> (210.1745, -12.5031)
  line L6444 (212.5746, -12.5031) -> (212.5746, -11.8381)
  line L6445 (212.5746, -11.8381) -> (212.3746, -11.8381)
  line L6446 (212.3746, -11.8381) -> (212.3746, -12.5031)
  line L6447 (212.3746, -12.5031) -> (212.5746, -12.5031)
  line L6448 (209.7745, -11.8381) -> (209.5745, -11.8381)
  line L6449 (209.7745, -12.5031) -> (209.7745, -11.8381)
  line L6450 (209.5745, -12.5031) -> (209.7745, -12.5031)
  line L6451 (209.5745, -11.8381) -> (209.5745, -12.5031)
  line L6452 (211.5745, -12.5031) -> (211.7745, -12.5031)
  line L6453 (211.5745, -11.8381) -> (211.5745, -12.5031)
  line L6454 (211.7745, -11.8381) -> (211.5745, -11.8381)
  line L6455 (211.7745, -12.5031) -> (211.7745, -11.8381)
  line L6456 (208.7744, -12.5031) -> (208.9744, -12.5031)
  line L6457 (208.7744, -11.8381) -> (208.7744, -12.5031)
  line L6458 (208.9744, -11.8381) -> (208.7744, -11.8381)
  line L6459 (208.9744, -12.5031) -> (208.9744, -11.8381)
  line L6460 (211.9745, -11.8381) -> (211.9745, -12.5031)
  line L6461 (212.1745, -12.5031) -> (212.1745, -11.8381)
  line L6462 (212.1745, -11.8381) -> (211.9745, -11.8381)
  line L6463 (211.9745, -12.5031) -> (212.1745, -12.5031)
  line L6464 (209.3744, -11.8381) -> (209.1744, -11.8381)
  line L6465 (209.1744, -12.5031) -> (209.3744, -12.5031)
  line L6466 (209.1744, -11.8381) -> (209.1744, -12.5031)
  line L6467 (209.3744, -12.5031) -> (209.3744, -11.8381)
  line L6468 (212.6745, -7.1629) -> (212.6745, -10.3629)
  line L6469 (209.4745, -7.1629) -> (212.6745, -7.1629)
  line L6470 (209.4745, -10.3629) -> (209.4745, -7.1629)
  line L6471 (212.6745, -10.3629) -> (209.4745, -10.3629)
  line L6472 (188.0514, -6.889) -> (188.0514, -7.131)
  line L6473 (188.0514, -6.559) -> (188.4214, -6.559)
  line L6474 (188.9014, -6.281) -> (188.1014, -6.281)
  line L6475 (188.9514, -6.331) -> (188.9014, -6.281)
  line L6476 (188.4214, -6.559) -> (188.4214, -6.889)
  line L6477 (188.0514, -6.331) -> (188.0514, -6.559)
  line L6478 (188.9514, -7.131) -> (188.9514, -6.331)
  line L6479 (188.1014, -6.281) -> (188.0514, -6.331)
  line L6480 (188.0514, -7.131) -> (188.1014, -7.181)
  line L6481 (188.9014, -7.181) -> (188.9514, -7.131)
  line L6482 (188.4214, -6.889) -> (188.0514, -6.889)
  line L6483 (188.1014, -7.181) -> (188.9014, -7.181)
  line L6484 (186.5114, -6.281) -> (186.4614, -6.331)
  line L6485 (186.4614, -6.331) -> (186.4614, -7.131)
  line L6486 (187.3114, -7.181) -> (187.3614, -7.131)
  line L6487 (187.3614, -7.131) -> (187.3614, -6.903)
  line L6488 (186.4614, -7.131) -> (186.5114, -7.181)
  line L6489 (187.3114, -6.281) -> (186.5114, -6.281)
  line L6490 (186.9914, -6.903) -> (186.9914, -6.573)
  line L6491 (186.9914, -6.573) -> (187.3614, -6.573)
  line L6492 (187.3614, -6.903) -> (186.9914, -6.903)
  line L6493 (187.3614, -6.331) -> (187.3114, -6.281)
  line L6494 (187.3614, -6.573) -> (187.3614, -6.331)
  line L6495 (186.5114, -7.181) -> (187.3114, -7.181)
  line L6496 (182.4194, -6.903) -> (182.4194, -6.573)
  line L6497 (182.7393, -6.281) -> (181.9393, -6.281)
  line L6498 (182.7894, -6.573) -> (182.7894, -6.331)
  line L6499 (181.9393, -7.181) -> (182.7393, -7.181)
  line L6500 (182.7393, -7.181) -> (182.7894, -7.131)
  line L6501 (182.7894, -7.131) -> (182.7894, -6.903)
  line L6502 (181.8894, -6.331) -> (181.8894, -7.131)
  line L6503 (182.7894, -6.903) -> (182.4194, -6.903)
  line L6504 (182.7894, -6.331) -> (182.7393, -6.281)
  line L6505 (181.9393, -6.281) -> (181.8894, -6.331)
  line L6506 (182.4194, -6.573) -> (182.7894, -6.573)
  line L6507 (181.8894, -7.131) -> (181.9393, -7.181)
  line L6508 (183.4794, -6.331) -> (183.4794, -6.559)
  line L6509 (184.3794, -7.131) -> (184.3794, -6.331)
  line L6510 (183.4794, -6.559) -> (183.8494, -6.559)
  line L6511 (183.8494, -6.889) -> (183.4794, -6.889)
  line L6512 (184.3294, -7.181) -> (184.3794, -7.131)
  line L6513 (184.3294, -6.281) -> (183.5294, -6.281)
  line L6514 (183.5294, -7.181) -> (184.3294, -7.181)
  line L6515 (183.4794, -7.131) -> (183.5294, -7.181)
  line L6516 (184.3794, -6.331) -> (184.3294, -6.281)
  line L6517 (183.5294, -6.281) -> (183.4794, -6.331)
  line L6518 (183.4794, -6.889) -> (183.4794, -7.131)
  line L6519 (183.8494, -6.559) -> (183.8494, -6.889)
  line L6520 (190.2693, -3.3138) -> (190.4706, -3.5151)
  line L6521 (189.4443, -4.8901) -> (189.4443, -3.7901)
  line L6522 (189.7193, -3.3138) -> (189.9943, -3.2401)
  line L6523 (189.9943, -3.2401) -> (190.2693, -3.3138)
  line L6524 (190.2693, -5.3664) -> (189.9943, -5.4401)
  line L6525 (189.518, -5.1651) -> (189.4443, -4.8901)
  line L6526 (190.5443, -4.8901) -> (190.4706, -5.1651)
  line L6527 (190.4706, -5.1651) -> (190.2693, -5.3664)
  line L6528 (190.4706, -3.5151) -> (190.5443, -3.7901)
  line L6529 (189.518, -3.5151) -> (189.7193, -3.3138)
  line L6530 (190.5443, -3.7901) -> (190.5443, -4.8901)
  line L6531 (189.4443, -3.7901) -> (189.518, -3.5151)
  line L6532 (189.9943, -5.4401) -> (189.7193, -5.3664)
  line L6533 (189.7193, -5.3664) -> (189.518, -5.1651)
  line L6534 (181.3545, -3.2401) -> (181.6295, -3.3138)
  line L6535 (181.8308, -5.1651) -> (181.6295, -5.3664)
  line L6536 (181.9045, -4.8901) -> (181.8308, -5.1651)
  line L6537 (181.9045, -3.7901) -> (181.9045, -4.8901)
  line L6538 (181.8308, -3.5151) -> (181.9045, -3.7901)
  line L6539 (181.0795, -3.3138) -> (181.3545, -3.2401)
  line L6540 (180.8781, -3.5151) -> (181.0795, -3.3138)
  line L6541 (181.6295, -5.3664) -> (181.3545, -5.4401)
  line L6542 (181.3545, -5.4401) -> (181.0795, -5.3664)
  line L6543 (180.8781, -5.1651) -> (180.8045, -4.8901)
  line L6544 (180.8045, -3.7901) -> (180.8781, -3.5151)
  line L6545 (181.6295, -3.3138) -> (181.8308, -3.5151)
  line L6546 (181.0795, -5.3664) -> (180.8781, -5.1651)
  line L6547 (180.8045, -4.8901) -> (180.8045, -3.7901)
  line L6548 (189.518, -0.865) -> (189.4443, -0.59)
  line L6549 (190.2693, -1.0663) -> (189.9943, -1.14)
  line L6550 (190.4706, 0.485) -> (190.5443, 0.21)
  line L6551 (189.4443, -0.59) -> (189.4443, 0.21)
  line L6552 (189.7193, -1.0663) -> (189.518, -0.865)
  line L6553 (189.518, 0.485) -> (189.7193, 0.6863)
  line L6554 (190.5443, -0.59) -> (190.4706, -0.865)
  line L6555 (190.4706, -0.865) -> (190.2693, -1.0663)
  line L6556 (189.9943, 0.76) -> (190.2693, 0.6863)
  line L6557 (190.5443, 0.21) -> (190.5443, -0.59)
  line L6558 (189.9943, -1.14) -> (189.7193, -1.0663)
  line L6559 (189.7193, 0.6863) -> (189.9943, 0.76)
  line L6560 (189.4443, 0.21) -> (189.518, 0.485)
  line L6561 (190.2693, 0.6863) -> (190.4706, 0.485)
  line L6562 (181.6295, -1.0663) -> (181.3545, -1.14)
  line L6563 (180.8045, 0.21) -> (180.8781, 0.485)
  line L6564 (181.8308, -0.865) -> (181.6295, -1.0663)
  line L6565 (181.0795, -1.0663) -> (180.8781, -0.865)
  line L6566 (180.8781, 0.485) -> (181.0795, 0.6863)
  line L6567 (181.9045, 0.21) -> (181.9045, -0.59)
  line L6568 (181.3545, 0.76) -> (181.6295, 0.6863)
  line L6569 (181.9045, -0.59) -> (181.8308, -0.865)
  line L6570 (181.6295, 0.6863) -> (181.8308, 0.485)
  line L6571 (180.8045, -0.59) -> (180.8045, 0.21)
  line L6572 (181.0795, 0.6863) -> (181.3545, 0.76)
  line L6573 (181.3545, -1.14) -> (181.0795, -1.0663)
  line L6574 (180.8781, -0.865) -> (180.8045, -0.59)
  line L6575 (181.8308, 0.485) -> (181.9045, 0.21)
  line L6576 (211.8854, -3.1359) -> (213.1854, -3.1359)
  line L6577 (211.8854, -3.4359) -> (211.8854, -3.1359)
  line L6578 (213.1854, -3.4359) -> (211.8854, -3.4359)
  line L6579 (213.1854, -3.1359) -> (213.1854, -3.4359)
  line L6580 (211.8854, -2.636) -> (213.1854, -2.636)
  line L6581 (213.1854, -2.936) -> (211.8854, -2.936)
  line L6582 (213.1854, -2.636) -> (213.1854, -2.936)
  line L6583 (211.8854, -2.936) -> (211.8854, -2.636)
  line L6584 (211.8854, -2.1361) -> (213.1854, -2.1361)
  line L6585 (211.8854, -2.4361) -> (211.8854, -2.1361)
  line L6586 (213.1854, -2.1361) -> (213.1854, -2.4361)
  line L6587 (213.1854, -2.4361) -> (211.8854, -2.4361)
  line L6588 (213.1854, -1.636) -> (213.1854, -1.936)
  line L6589 (211.8854, -1.936) -> (211.8854, -1.636)
  line L6590 (211.8854, -1.636) -> (213.1854, -1.636)
  line L6591 (213.1854, -1.936) -> (211.8854, -1.936)
  line L6592 (211.8854, -1.4359) -> (211.8854, -1.1359)
  line L6593 (213.1854, -1.1359) -> (213.1854, -1.4359)
  line L6594 (213.1854, -1.4359) -> (211.8854, -1.4359)
  line L6595 (211.8854, -1.1359) -> (213.1854, -1.1359)
  line L6596 (207.1854, -1.1361) -> (208.4854, -1.1361)
  line L6597 (208.4854, -1.4361) -> (207.1854, -1.4361)
  line L6598 (208.4854, -1.1361) -> (208.4854, -1.4361)
  line L6599 (207.1854, -1.4361) -> (207.1854, -1.1361)
  line L6600 (207.1854, -1.936) -> (207.1854, -1.636)
  line L6601 (207.1854, -1.636) -> (208.4854, -1.636)
  line L6602 (208.4854, -1.636) -> (208.4854, -1.936)
  line L6603 (208.4854, -1.936) -> (207.1854, -1.936)
  line L6604 (208.4854, -2.1359) -> (208.4854, -2.4359)
  line L6605 (207.1854, -2.4359) -> (207.1854, -2.1359)
  line L6606 (207.1854, -2.1359) -> (208.4854, -2.1359)
  line L6607 (208.4854, -2.4359) -> (207.1854, -2.4359)
  line L6608 (207.1854, -2.936) -> (207.1854, -2.636)
  line L6609 (207.1854, -2.636) -> (208.4854, -2.636)
  line L6610 (208.4854, -2.636) -> (208.4854, -2.936)
  line L6611 (208.4854, -2.936) -> (207.1854, -2.936)
  line L6612 (208.4854, -3.4361) -> (207.1854, -3.4361)
  line L6613 (207.1854, -3.1361) -> (208.4854, -3.1361)
  line L6614 (207.1854, -3.4361) -> (207.1854, -3.1361)
  line L6615 (208.4854, -3.1361) -> (208.4854, -3.4361)
  line L6616 (138.2252, -77.2806) -> (138.2252, -76.4406)
  line L6617 (138.2252, -76.4406) -> (139.1352, -76.4406)
  line L6618 (139.1352, -77.2806) -> (138.2252, -77.2806)
  line L6619 (139.1352, -76.4406) -> (139.1352, -77.2806)
  line L6620 (142.4454, -76.4406) -> (142.4454, -77.2806)
  line L6621 (141.5353, -77.2806) -> (141.5353, -76.4406)
  line L6622 (141.5353, -76.4406) -> (142.4454, -76.4406)
  line L6623 (142.4454, -77.2806) -> (141.5353, -77.2806)
  line L6624 (138.2252, -20.105) -> (138.2252, -19.265)
  line L6625 (138.2252, -19.265) -> (139.1352, -19.265)
  line L6626 (139.1352, -19.265) -> (139.1352, -20.105)
  line L6627 (139.1352, -20.105) -> (138.2252, -20.105)
  line L6628 (141.5353, -20.105) -> (141.5353, -19.265)
  line L6629 (142.4454, -19.265) -> (142.4454, -20.105)
  line L6630 (141.5353, -19.265) -> (142.4454, -19.265)
  line L6631 (142.4454, -20.105) -> (141.5353, -20.105)
  line L6632 (138.2252, -39.1551) -> (138.2252, -38.3151)
  line L6633 (139.1352, -38.3151) -> (139.1352, -39.1551)
  line L6634 (139.1352, -39.1551) -> (138.2252, -39.1551)
  line L6635 (138.2252, -38.3151) -> (139.1352, -38.3151)
  line L6636 (141.5353, -38.3151) -> (142.4454, -38.3151)
  line L6637 (142.4454, -38.3151) -> (142.4454, -39.1551)
  line L6638 (142.4454, -39.1551) -> (141.5353, -39.1551)
  line L6639 (141.5353, -39.1551) -> (141.5353, -38.3151)
  line L6640 (139.1352, -57.3778) -> (139.1352, -58.2178)
  line L6641 (138.2252, -58.2178) -> (138.2252, -57.3778)
  line L6642 (139.1352, -58.2178) -> (138.2252, -58.2178)
  line L6643 (138.2252, -57.3778) -> (139.1352, -57.3778)
  line L6644 (142.4454, -57.3778) -> (142.4454, -58.2178)
  line L6645 (141.5353, -57.3778) -> (142.4454, -57.3778)
  line L6646 (142.4454, -58.2178) -> (141.5353, -58.2178)
  line L6647 (141.5353, -58.2178) -> (141.5353, -57.3778)
  line L6648 (157.2752, -20.105) -> (157.2752, -19.265)
  line L6649 (157.2752, -19.265) -> (158.1853, -19.265)
  line L6650 (158.1853, -19.265) -> (158.1853, -20.105)
  line L6651 (158.1853, -20.105) -> (157.2752, -20.105)
  line L6652 (161.4954, -20.105) -> (160.5854, -20.105)
  line L6653 (160.5854, -20.105) -> (160.5854, -19.265)
  line L6654 (160.5854, -19.265) -> (161.4954, -19.265)
  line L6655 (161.4954, -19.265) -> (161.4954, -20.105)
  line L6656 (157.2752, -77.2806) -> (157.2752, -76.4406)
  line L6657 (158.1853, -77.2806) -> (157.2752, -77.2806)
  line L6658 (157.2752, -76.4406) -> (158.1853, -76.4406)
  line L6659 (158.1853, -76.4406) -> (158.1853, -77.2806)
  line L6660 (161.4954, -77.2806) -> (160.5854, -77.2806)
  line L6661 (160.5854, -76.4406) -> (161.4954, -76.4406)
  line L6662 (160.5854, -77.2806) -> (160.5854, -76.4406)
  line L6663 (161.4954, -76.4406) -> (161.4954, -77.2806)
  line L6664 (157.2752, -57.3778) -> (158.1853, -57.3778)
  line L6665 (158.1853, -57.3778) -> (158.1853, -58.2178)
  line L6666 (157.2752, -58.2178) -> (157.2752, -57.3778)
  line L6667 (158.1853, -58.2178) -> (157.2752, -58.2178)
  line L6668 (160.5854, -58.2178) -> (160.5854, -57.3778)
  line L6669 (161.4954, -57.3778) -> (161.4954, -58.2178)
  line L6670 (160.5854, -57.3778) -> (161.4954, -57.3778)
  line L6671 (161.4954, -58.2178) -> (160.5854, -58.2178)
  line L6672 (157.2752, -38.3151) -> (158.1853, -38.3151)
  line L6673 (158.1853, -39.1551) -> (157.2752, -39.1551)
  line L6674 (158.1853, -38.3151) -> (158.1853, -39.1551)
  line L6675 (157.2752, -39.1551) -> (157.2752, -38.3151)
  line L6676 (160.5854, -38.3151) -> (161.4954, -38.3151)
  line L6677 (161.4954, -39.1551) -> (160.5854, -39.1551)
  line L6678 (161.4954, -38.3151) -> (161.4954, -39.1551)
  line L6679 (160.5854, -39.1551) -> (160.5854, -38.3151)
  line L6680 (176.3253, -19.265) -> (177.2353, -19.265)
  line L6681 (177.2353, -20.105) -> (176.3253, -20.105)
  line L6682 (177.2353, -19.265) -> (177.2353, -20.105)
  line L6683 (176.3253, -20.105) -> (176.3253, -19.265)
  line L6684 (180.5454, -19.265) -> (180.5454, -20.105)
  line L6685 (179.6354, -20.105) -> (179.6354, -19.265)
  line L6686 (180.5454, -20.105) -> (179.6354, -20.105)
  line L6687 (179.6354, -19.265) -> (180.5454, -19.265)
  line L6688 (177.2353, -76.4406) -> (177.2353, -77.2806)
  line L6689 (176.3253, -77.2806) -> (176.3253, -76.4406)
  line L6690 (177.2353, -77.2806) -> (176.3253, -77.2806)
  line L6691 (176.3253, -76.4406) -> (177.2353, -76.4406)
  line L6692 (180.5454, -76.4406) -> (180.5454, -77.2806)
  line L6693 (179.6354, -76.4406) -> (180.5454, -76.4406)
  line L6694 (179.6354, -77.2806) -> (179.6354, -76.4406)
  line L6695 (180.5454, -77.2806) -> (179.6354, -77.2806)
  line L6696 (177.2353, -57.3778) -> (177.2353, -58.2178)
  line L6697 (177.2353, -58.2178) -> (176.3253, -58.2178)